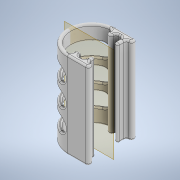
# Autodesk Inventor part: CableCap
Saved by Autodesk Inventor 2020 (Build 240168000, 168)
## iProperties
Created: 2020-07-28
Part Number: CableCap
Material: Generic
Document SubType Name: Modeling
Designer: maple
Density: 1 g/cm^3
Appearance: Default
Author: maple
Autodesk Inventor part; units mm, degrees
ref_plane "YZ Plane" through (0, 0, 0) normal (1, 0, 0) x (0, 1, 0)
ref_plane "XZ Plane" through (0, 0, 0) normal (0, 1, 0) x (-1, 0, 0)
sketch "Sketch1" plane through (0, 0, 0) normal (0, 1, 0) x (-1, 0, 0)
  line L0 (0, 0) -> (2, 0)
  line L1 (2, 0) -> (2, -3)
  line L2 (2, -3) -> (0, -3)
  line L3 (0, -3) -> (0, 0)
  line L4 (0, 0) -> (0, -20)
  line L5 (0, -20) -> (2, -20)
  line L6 (2, -20) -> (2, -16)
  line L7 (2, -16) -> (0, -16)
  line L8 (0, -16) -> (0, -20)
  line L9 (0, 0) -> (2, 0)
  line L10 (2, 0) -> (2, 1)
  line L11 (2, 1) -> (0, 1)
  line L12 (0, 1) -> (0, 0)
  line L13 (0, -20) -> (2, -20)
  line L14 (2, -20) -> (2, -21)
  line L15 (2, -21) -> (0, -21)
  line L16 (0, -21) -> (0, -20)
  line L17 (0, 1) -> (6, 1)
  line L18 (6, 1) -> (6, 4)
  line L19 (6, 4) -> (0, 4)
  line L20 (0, 4) -> (0, 1)
  line L21 (0, -21) -> (6, -21)
  line L22 (6, -21) -> (6, -24)
  line L23 (6, -24) -> (0, -24)
  line L24 (0, -24) -> (0, -21)
  line L25 (6, 4) -> (9, 4)
  line L26 (9, 4) -> (9, -1.5)
  line L27 (9, -1.5) -> (6, -1.5)
  line L28 (6, -1.5) -> (6, 4)
  line L29 (6, -24) -> (9, -24)
  line L30 (9, -24) -> (9, -18.4882)
  line L31 (9, -18.4882) -> (6, -18.4882)
  line L32 (6, -18.4882) -> (6, -24)
  line L33 (0, 4) -> (-3, 4)
  line L34 (-3, 4) -> (-3, 1)
  line L35 (-3, 1) -> (0, 1)
  line L36 (0, 1) -> (0, 4)
  line L37 (0, -21) -> (-3, -21)
  line L38 (-3, -21) -> (-3, -24)
  line L39 (-3, -24) -> (0, -24)
  line L40 (0, -24) -> (0, -21)
  line L41 (9, 4) -> (9, -24)
  line L42 (9, -10) -> (23, -10)
  arc A0 (9, -24) -> (9, 4) centre (9, -10) ccw
  line L43 (9, 4) -> (9, 2)
  line L44 (9, -24) -> (9, -22)
  arc A1 (9, -22) -> (9, 2) centre (9, -10) ccw
  dimension "d0" = 2
  dimension "d1" = 3
  dimension "d2" = 20
  dimension "d3" = 2
  dimension "d4" = 4
  dimension "d5" = 2
  dimension "d6" = 1
  dimension "d7" = 2
  dimension "d8" = 1
  dimension "d9" = 6
  dimension "d10" = 3
  dimension "d11" = 6
  dimension "d12" = 3
  dimension "d13" = 3
  dimension "d14" = 3
  dimension "d15" = 5.5118
  dimension "d16" = 3
  dimension "d17" = 3
  dimension "d18" = 3
  dimension "d19" = 3
  dimension "d20" = 14
  dimension "d21" = 2
  dimension "d22" = 2
  constraints: 90 end point, 20 parallel, 11 horizontal, 10 perpendicular, 5 point on circle, 2 centre point, 2 point on line, 1 midpoint, 1 vertical
  measures "d0" distance of L1.end L2.end
  measures "d1" distance of L0.end L1.end
  measures "d2" distance of L0.start L4.end
  measures "d3" distance of L7.end L6.end
  measures "d4" distance of L6.end L5.end
  measures "d5" distance of L11.end L10.end
  measures "d6" distance of L10.end L9.end
  measures "d7" distance of L14.end L15.end
  measures "d8" distance of L13.end L14.end
  measures "d9" distance of L19.end L18.end
  measures "d10" distance of L18.end L17.end
  measures "d11" distance of L22.end L23.end
  measures "d12" distance of L21.end L22.end
  measures "d13" distance of L26.end L27.end
  measures "d14" distance of L31.end L30.end
  measures "d15" distance of L30.end L29.end
  measures "d16" distance of L35.end L34.end
  measures "d17" distance of L34.end L33.end
  measures "d18" distance of L39.end L38.end
  measures "d19" distance of L38.end L37.end
  measures "d20" distance of L42.start L42.end
  measures "d21" distance of L25.end L43.end
  measures "d22" distance of L29.end L44.end
extrude "Extrusion1" add sketch "Sketch1" along normal blind 50 contours L12 L11 L10 L0 | L0 L1 L2 L3 | L20 L19 L18 L17 L11 | L35 L34 L33 L20 | L7 L6 L5 L4 | L18 L25 L26 L27 L28 | L5 L14 L15 L16 | L15 L21 L22 L23 L24 | L24 L39 L38 L37 | A0 L42 A1 L26 | A0 L30 A1 L42 | L32 L31 L30 L29 L22
fillet "Fillet1" radius 1.5 8 edges at (-9, 25, -1.5) (-6, 25, -1.5) (-9, 25, -18.4882) (-6, 25, -18.4882) (3, 25, 4) (3, 25, 1) (3, 25, -21) (3, 25, -24)
fillet "Fillet2" radius 1 4 edges at (-2, 25, -3) (0, 25, -3) (-2, 25, -16) (0, 25, -16)
fillet "Fillet3" radius 1.5 8 edges at (-6, 25, 1) (-2, 25, 1) (-6, 25, -21) (-2, 25, -21) (0, 25, 1) (0, 25, -21) (-9, 25, 2) (-9, 25, -22)
fillet "Fillet4" radius 1 54 edges at (-3, 50, 4) (-23, 50, -10) (-3, 50, -24) (2.5607, 50, -21.4393) (1.5, 50, -21) (0, 50, -18.25) (-1.7071, 50, -16.2929) (-2, 50, -18.25) (-2.4393, 50, -20.5607) (-4.02, 50, -21) (-5.5106, 50, -20.6437) (-8.5607, 50, -18.9275) (-9, 50, -20.1903) (-9.518, 50, -21.5262) (-21, 50, -10) (-9.518, 50, 1.5262) (-9, 50, 0.1962) (-8.5607, 50, -1.0607) (-5.5102, 50, 0.6456) (-4.021, 50, 1) (-2.4393, 50, 0.5607) (-2, 50, -1.25) (-1.7071, 50, -2.7071) (0, 50, -1.25) (1.5, 50, 1) (3, 50, 2.5) (2.5607, 50, 3.5607) (-3, 0, 4) (3, 0, 2.5) (2.5607, 0, 3.5607) (1.5, 0, 1) (0, 0, -1.25) (-1.7071, 0, -2.7071) (-2, 0, -1.25) (-2.4393, 0, 0.5607) (-4.021, 0, 1) (-5.5102, 0, 0.6456) (-8.5607, 0, -1.0607) (-9, 0, 0.1962) (-9.518, 0, 1.5262) (-21, 0, -10) (-9.518, 0, -21.5262) (-9, 0, -20.1903) (-8.5607, 0, -18.9275) (-5.5106, 0, -20.6437) (-4.02, 0, -21) (-2.4393, 0, -20.5607) (-2, 0, -18.25) (-1.7071, 0, -16.2929) (0, 0, -18.25) (1.5, 0, -21) (2.5607, 0, -21.4393) (-3, 0, -24) (-23, 0, -10)
ref_plane "Work Plane1" through (0, 0, -9.525) normal (0, 0, 1) x (1, 0, 0)
sketch "Sketch2" plane through (0, 0, -9.525) normal (0, 0, 1) x (1, 0, 0)
  line L0 (-9, 0) -> (-22, 0) projected
  line L1 (-14.3128, 0) -> (-14.3128, 50)
  line L2 (-14.3128, 0) -> (-14.3128, 12.5)
  line L3 (-14.3128, 12.5) -> (-14.3128, 25)
  line L4 (-14.3128, 25) -> (-14.3128, 37.5)
  line L5 (-14.3128, 37.5) -> (-14.3128, 50)
  circle A0 centre (-14.3128, 12.5) radius 4
  circle A1 centre (-14.3128, 25) radius 4
  circle A2 centre (-14.3128, 37.5) radius 4
  line L6 (-14.3128, 8.5) -> (-25.7761, 8.5)
  line L7 (-25.7761, 8.5) -> (-25.7761, 16.5)
  line L8 (-25.7761, 16.5) -> (-14.3128, 16.5)
  line L9 (-14.3128, 16.5) -> (-14.3128, 8.5)
  line L10 (-14.3128, 21) -> (-25.7761, 21)
  line L11 (-25.7761, 21) -> (-25.7761, 29)
  line L12 (-25.7761, 29) -> (-14.3128, 29)
  line L13 (-14.3128, 29) -> (-14.3128, 21)
  line L14 (-14.3128, 33.5) -> (-25.7761, 33.5)
  line L15 (-25.7761, 33.5) -> (-25.7761, 41.5)
  line L16 (-25.7761, 41.5) -> (-14.3128, 41.5)
  line L17 (-14.3128, 41.5) -> (-14.3128, 33.5)
  point P0 (0, 0)
  dimension "d34" = 8
  dimension "d35" = 8
  dimension "d36" = 8
  dimension "d30" = 50
  dimension "d31" = 12.5
  dimension "d32" = 12.5
  dimension "d33" = 12.5
  constraints: 34 end point, 8 point on line, 6 parallel, 3 coincident, 3 horizontal, 3 perpendicular, 1 collinear, 1 midpoint, 1 vertical, 9 other
  measures "d30" distance of L1.start L1.end
  measures "d31" distance of L1.start L2.end
  measures "d32" distance of L2.end L3.end
  measures "d33" distance of L3.end L4.end
extrude "Extrusion2" cut sketch "Sketch2" along normal mid plane 50
fillet "Fillet5" radius 0.8 36 edges at (-12.1209, 34.154, 1.5871) (-10.3128, 37.5, 1.8806) (-12.1209, 40.846, 1.5871) (-21, 41.5, -10) (-12.1209, 40.846, -21.5871) (-10.3128, 37.5, -21.8806) (-12.1209, 34.154, -21.5871) (-21, 33.5, -10) (-10.3128, 37.5006, 3.9383) (-10.3128, 37.5006, -23.9383) (-23, 41.5, -10) (-23, 33.5, -10) (-12.1209, 21.654, 1.5871) (-10.3128, 25, 1.8806) (-12.1209, 28.346, 1.5871) (-21, 29, -10) (-12.1209, 28.346, -21.5871) (-10.3128, 25, -21.8806) (-12.1209, 21.654, -21.5871) (-21, 21, -10) (-10.3128, 25.0006, 3.9383) (-10.3128, 25.0006, -23.9383) (-23, 29, -10) (-23, 21, -10) (-12.1209, 9.154, 1.5871) (-10.3128, 12.5, 1.8806) (-12.1209, 15.846, 1.5871) (-21, 16.5, -10) (-12.1209, 15.846, -21.5871) (-10.3128, 12.5, -21.8806) (-12.1209, 9.154, -21.5871) (-21, 8.5, -10) (-10.3128, 12.5006, 3.9383) (-10.3128, 12.5006, -23.9383) (-23, 16.5, -10) (-23, 8.5, -10)
body "Solid1"
